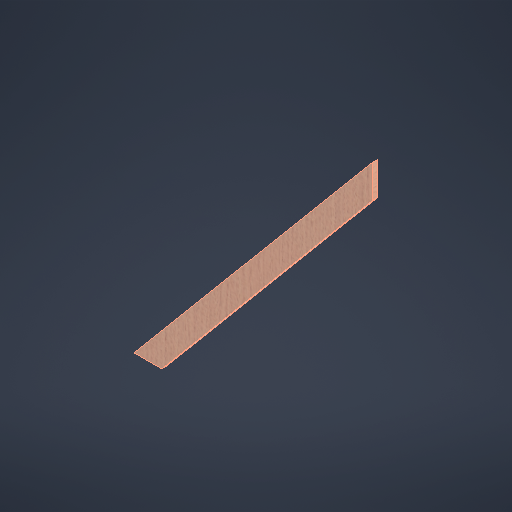
# Autodesk Inventor part: SUPPORTS_TREBUCHET
Saved by Autodesk Inventor 2026.2 (Build 302298010, 298A)
## iProperties
Created: 2026-02-18
Part Number: SUPPORTS_TREBUCHET
Material: Wood (Oak)
Document SubType Name: Modeling
Designer: 4aida
Density: 0.76 g/cm^3
Appearance: White Oak - Natural Medium Gloss
Author: 4aida
Autodesk Inventor part; units mm, degrees
ref_plane "YZ Plane" through (0, 0, 0) normal (1, 0, 0) x (0, 1, 0)
ref_plane "XZ Plane" through (0, 0, 0) normal (0, 1, 0) x (-1, 0, 0)
ref_plane "XY Plane" through (0, 0, 0) normal (0, 0, 1) x (1, 0, 0)
sketch "Sketch1" plane through (0, 0, 0) normal (0, 0, 1) x (1, 0, 0)
  line L0 (201.8785, 270.226) -> (-226.7465, -240.5894)
  line L1 (-226.7465, -240.5894) -> (-177.0105, -240.5894)
  line L2 (-177.0105, -240.5894) -> (201.8785, 210.9529)
  line L3 (201.8785, 210.9529) -> (201.8785, 270.226)
  line L4 (-12.434, 14.8183) -> (12.434, -14.8183) construction
  point P0 (0, 0)
  point P1 (0, 0)
  dimension "d0" = 50
  dimension "d1" = 38.1
  dimension "d2" = 428.625
  constraints: 10 end point, 3 midpoint, 1 coincident, 1 horizontal, 1 parallel, 1 perpendicular
  measures "d0" angle of L1 L2
  measures "d1" distance between parallel lines of L0 L2
  measures "d2" distance from line of L3 L0.end
extrude "Extrusion1" add sketch "Sketch1" along normal blind 9.525
body "Solid1"
